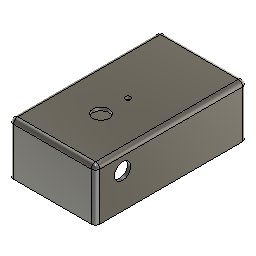
Upper housing v9 (Autodesk Fusion 360 design; units mm, degrees)
Autodesk Fusion 360 part; units mm, degrees
sketch "Sketch1" plane through (0, 0, 0) normal (0, 0, 1) x (1, 0, 0)
  line L0 (0, 0) -> (80, 0)
  line L1 (80, 0) -> (80, 140)
  line L2 (80, 140) -> (0, 140)
  line L3 (0, 140) -> (0, 0)
  line L4 (40, 140) -> (40, 0) construction
  circle A0 centre (40, 45) radius 7.5
  line L5 (5, 5) -> (75, 5) construction
  line L6 (75, 5) -> (75, 135) construction
  line L7 (75, 135) -> (5, 135) construction
  line L8 (5, 135) -> (5, 5) construction
  circle A1 centre (75, 135) radius 1.65
  circle A2 centre (5, 135) radius 1.65
  circle A3 centre (75, 5) radius 1.65
  circle A4 centre (5, 5) radius 1.65
  circle A5 centre (75, 5) radius 3.15
  circle A6 centre (5, 5) radius 3.15
  circle A7 centre (5, 135) radius 3.15
  circle A8 centre (75, 135) radius 3.65
  circle A9 centre (40, 70) radius 2.5
  dimension "d1" = 80
  dimension "d2" = 140
  dimension "d3" = 15
  dimension "d13" = -5
  dimension "d14" = 3.3
  dimension "d15" = 3.3
  dimension "d16" = 3.3
  dimension "d17" = 3.3
  dimension "d18" = 1.5
  dimension "d19" = 1.5
  dimension "d20" = 1.5
  dimension "d21" = 2
  dimension "d38" = 45
  dimension "d40" = 5
  dimension "d41" = 25
  constraint horizontal L0
  constraint vertical L1
  constraint horizontal L2
  constraint vertical L3
  constraint coincident L0.start L3.end
  constraint midpoint L2 L4.start
  constraint midpoint L0 L4.end
  constraint coincident L4 A0.centre
  constraint coincident L6.end L7.start
  constraint coincident L7.end L8.start
  constraint coincident L5.end L6.start
  constraint coincident L5.start L8.end
  constraint coincident L4 A9.centre
  measures "d1" distance of L0.start L0.end
  measures "d2" distance of L0.start L2.end
  measures "d3" diameter of A0
  measures "d14" diameter of A1
  measures "d15" diameter of A2
  measures "d16" diameter of A3
  measures "d17" diameter of A4
  measures "d38" distance of L0 A0.centre
  measures "d40" diameter of A9
  measures "d41" distance of A0.centre A9.centre
extrude "Extrude1" add sketch "Sketch1" along normal blind 48 contours L0 L1 L2 L3 | A0 | A1 | A2 | A3 | A4 | A5 | A6 | A7 | A8 | A9
shell "Shell1" thickness 3 removed faces 1 at (26.6667, 46.6667, 0)
extrude "Footswitch hole" cut sketch "Sketch1" along normal up to surface (48 mm away) contours A0 | A9
sketch "Sketch3" plane through (0, 0, 0) normal (-1, 0, 0) x (0, -1, 0)
  line L0 (-140, 0) -> (0, 0)
  line L1 (0, 0) -> (0, 48)
  line L2 (0, 48) -> (-140, 48)
  line L3 (-140, 48) -> (-140, 0)
  line L4 (-130, 32) -> (0, 32) construction
  circle A0 centre (-25, 32) radius 7.5
  dimension "d28" = 15
  dimension "d37" = 25
  dimension "d39" = 16
  constraint coincident L4 A0.centre
  measures "d28" diameter of A0
  measures "d37" distance of L1 A0.centre
  measures "d39" distance of L2 L4
extrude "Extrude5" cut sketch "Sketch3" against normal up to surface (80 mm away) contours A0
fillet "Fillet1" radius 4 8 edges at (0, 0, 24) (3, 3, 22.5) (80, 0, 24) (77, 3, 22.5) (0, 140, 24) (3, 137, 22.5) (77, 137, 22.5) (80, 140, 24)
fillet "Fillets" radius 4 8 edges at (1.1716, 1.1716, 48) (40, 0, 48) (78.8284, 1.1716, 48) (80, 70, 48) (78.8284, 138.8284, 48) (40, 140, 48) (1.1716, 138.8284, 48) (0, 70, 48)
extrude "Extrude3" add sketch "Sketch1" along normal up to surface (45 mm away) contours A5 | A6 | A7 | A8
extrude "Extrude4" cut sketch "Sketch1" along normal up to surface (45 mm away) contours A1 | A2 | A3 | A4
fillet "Fillet3" radius 3 8 edges at (72.5664, 3, 22.5) (77, 7.4336, 22.5) (3, 7.4336, 22.5) (7.4336, 3, 22.5) (7.4336, 137, 22.5) (3, 132.5664, 22.5) (77, 131.9467, 22.5) (71.9467, 137, 22.5)
sketch "Sketch4" plane through (0, 140, 0) normal (0, 1, 0) x (-1, 0, 0)
  line L0 (-4, 44) -> (-76, 44)
  line L1 (-76, 44) -> (-76, 0)
  line L2 (-76, 0) -> (-4, 0)
  line L3 (-4, 0) -> (-4, 44)
  line L4 (-30, 18.7772) -> (-50, 18.7772)
  line L5 (-50, 18.7772) -> (-50, 5.7772)
  line L6 (-50, 5.7772) -> (-30, 5.7772)
  line L7 (-30, 5.7772) -> (-30, 18.7772)
  line L8 (-40, 44) -> (-40, 0) construction
  line L9 (-30, 12.2772) -> (-65, 12.2772) construction
  circle A0 centre (-65, 12.2772) radius 2.5
  dimension "d31" = 20
  dimension "d32" = 13
  dimension "d42" = 5
  dimension "d43" = 15
  constraint horizontal L4
  constraint vertical L5
  constraint horizontal L6
  constraint vertical L7
  constraint midpoint L0 L8.start
  constraint midpoint L2 L8.end
  constraint symmetric L5 L7 L8
  constraint midpoint L7 L9.start
  constraint perpendicular L7 L9
  constraint coincident L9.end A0.centre
  measures "d31" distance of L4.start L4.end
  measures "d32" distance of L4.start L6.end
  measures "d42" diameter of A0
  measures "d43" distance of L5 L9.end
extrude "Extrude6" cut sketch "Sketch4" against normal up to surface (3 mm away) contours L4 L5 L6 L7 | A0
equation "d38 = 35 mm + 10 mm"
